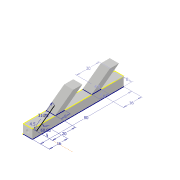
# Autodesk Inventor part: MineralStop1.25x60
Saved by Autodesk Inventor 2018 (Build 220112000, 112)
## iProperties
Created: 2018-12-12
Part Number: MineralStop1.25x60
Material: Generic
Document SubType Name: Modeling
Designer: ball
Density: 1 g/cm^3
Appearance: Default
Author: ball
Autodesk Inventor part; units mm, degrees
ref_plane "YZ Plane" through (0, 0, 0) normal (1, 0, 0) x (0, 1, 0)
ref_plane "XZ Plane" through (0, 0, 0) normal (0, 1, 0) x (-1, 0, 0)
ref_plane "XY Plane" through (0, 0, 0) normal (0, 0, 1) x (1, 0, 0)
sketch "Sketch1" plane through (0, 0, 0) normal (0, 1, 0) x (-1, 0, 0)
  line L0 (0, 0) -> (-8, 0)
  line L1 (-8, 0) -> (-8, -80)
  line L2 (-8, -80) -> (0, -80)
  line L3 (0, -80) -> (0, 0)
  circle A0 centre (-4, -16) radius 2.25
  circle A1 centre (-4, -64) radius 2.25
  dimension "d0" = 8
  dimension "d1" = 80
  dimension "d6" = 4.5
  dimension "d7" = 4.5
  dimension "d26" = 16
  dimension "d27" = 16
  constraints: 8 end point, 2 centre point, 2 parallel, 1 horizontal, 1 perpendicular
  measures "d0" distance of L2.end L1.end
  measures "d1" distance of L1.end L0.end
  measures "d6" diameter of A0
  measures "d7" diameter of A1
  measures "d26" distance from line of L0 A0.centre
  measures "d27" distance from line of L2 A1.centre
extrude "Extrusion1" [suppressed]
extrude "Extrusion2" add sketch "Sketch1" along normal blind 8
sketch "Sketch2" plane through (0, 0, 0) normal (0, 0, 1) x (1, 0, 0)
  circle A0 centre (4, 4) radius 1.35
  point P0 (0, 0)
  dimension "d10" = 2.7
  constraints: 1 centre point
  measures "d10" diameter of A0
hole "Hole1" at (4, 4, 0) direction (0, 0, -1) diameter 2.7 depth 10
sketch "Sketch3" plane through (8, 0, -80) normal (0, 0, -1) x (-1, 0, 0)
  circle A0 centre (4, 4) radius 1.35
  point P0 (8, 0)
  dimension "d18" = 2.7
  constraints: 1 centre point
  measures "d18" diameter of A0
hole "Hole2" at (4, 4, -80) direction (0, 0, 1) diameter 2.7 depth 10
sketch "Sketch5" plane through (0, 0, 0) normal (0, 0, 1) x (1, 0, 0)
  line L0 (11.5271, 8) -> (27.4021, 35.4963)
  line L1 (11.5271, 8) -> (43.2771, 8) construction
  point P0 (0, 0)
  dimension "d33" = 31.75
  dimension "d34" = 60
  constraints: 4 end point, 1 equal length, 1 horizontal
  measures "d33" distance of L0.start L0.end
  measures "d34" angle of L1 L0
sketch "Sketch4" plane through (0, 8, 0) normal (0, 1, 0) x (1, 0, 0)
  line L0 (0, 80) -> (0, 0) projected
  line L1 (8, 0) -> (8, 80) projected
  line L2 (0, 28) -> (8, 28)
  line L3 (8, 28) -> (8, 20)
  line L4 (8, 20) -> (0, 20)
  line L5 (0, 20) -> (0, 28)
  line L6 (0, 0) -> (8, 0) projected
  line L7 (0, 60) -> (8, 60)
  line L8 (8, 60) -> (8, 52)
  line L9 (8, 52) -> (0, 52)
  line L10 (0, 52) -> (0, 60)
  line L11 (8, 80) -> (0, 80) projected
  dimension "d28" = 8
  dimension "d29" = 20
  dimension "d30" = 8
  dimension "d31" = 20
  constraints: 16 end point, 4 parallel, 4 point on line, 2 horizontal, 2 perpendicular
  measures "d28" distance of L2.end L3.end
  measures "d29" distance between parallel lines of L6 L4
  measures "d30" distance of L7.end L8.end
  measures "d31" distance between parallel lines of L11 L7
sweep "Sweep1" add profiles "Sketch4" path "Sketch5" contours L2 L1 L4 L0
sweep "Sweep2" add profiles "Sketch4" path "Sketch5" contours L7 L1 L9 L0
body "Solid1"
